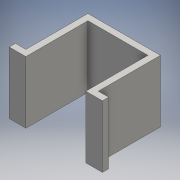
# Autodesk Inventor part: imu_case_2
Saved by Autodesk Inventor 2016 (Build 200138000, 138)
## iProperties
Created: 2015-11-15
Part Number: imu_case_2
Material: Generic
Document SubType Name: Modeling
Designer: Qiuyang
Density: 1 g/cm^3
Appearance: Default
Author: Qiuyang
Autodesk Inventor part; units mm, degrees
ref_plane "YZ Plane" through (0, 0, 0) normal (1, 0, 0) x (0, 1, 0)
ref_plane "XZ Plane" through (0, 0, 0) normal (0, 1, 0) x (-1, 0, 0)
ref_plane "XY Plane" through (0, 0, 0) normal (0, 0, 1) x (1, 0, 0)
sketch "Sketch2" plane through (0, 0, 0) normal (0, 0, 1) x (1, 0, 0)
  line L0 (0, 0) -> (5, 0)
  line L1 (5, 0) -> (5, 3)
  line L2 (5, 3) -> (0, 3)
  line L3 (0, 3) -> (0, 0)
  line L4 (5, 0) -> (8, 0)
  line L5 (8, 0) -> (8, 30)
  line L6 (8, 30) -> (5, 30)
  line L7 (5, 30) -> (5, 0)
  line L8 (5, 30) -> (40, 30)
  line L9 (40, 30) -> (40, 33)
  line L10 (40, 33) -> (5, 33)
  line L11 (5, 33) -> (5, 30)
  line L12 (40, 30) -> (37, 30)
  line L13 (37, 30) -> (37, 0)
  line L14 (37, 0) -> (40, 0)
  line L15 (40, 0) -> (40, 30)
  line L16 (40, 0) -> (45, 0)
  line L17 (45, 0) -> (45, 3)
  line L18 (45, 3) -> (40, 3)
  line L19 (40, 3) -> (40, 0)
  dimension "d0" = 5
  dimension "d1" = 3
  dimension "d2" = 3
  dimension "d3" = 30
  dimension "d4" = 35
  dimension "d5" = 3
  dimension "d6" = 3
  dimension "d7" = 30
  dimension "d8" = 5
  dimension "d9" = 3
  constraints: 40 end point, 10 parallel, 5 horizontal, 5 perpendicular
  measures "d0" distance of L2.end L1.end
  measures "d1" distance of L1.end L0.end
  measures "d2" distance of L6.end L5.end
  measures "d3" distance of L5.end L4.end
  measures "d4" distance of L10.end L9.end
  measures "d5" distance of L9.end L8.end
  measures "d6" distance of L14.end L13.end
  measures "d7" distance of L13.end L12.end
  measures "d8" distance of L18.end L17.end
  measures "d9" distance of L17.end L16.end
extrude "Extrusion1" add sketch "Sketch2" along normal blind 30
body "Solid1"
